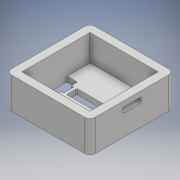
# Autodesk Inventor part: Part4
Saved by Autodesk Inventor 2018 (Build 220112000, 112)
## iProperties
Created: 2019-01-10
Part Number: Part4
Material: Generic
Document SubType Name: Modeling
Designer: USER
Density: 1 g/cm^3
Appearance: Default
Author: USER
Autodesk Inventor part; units mm, degrees
ref_plane "YZ Plane" through (0, 0, 0) normal (1, 0, 0) x (0, 1, 0)
ref_plane "XZ Plane" through (0, 0, 0) normal (0, 1, 0) x (-1, 0, 0)
ref_plane "XY Plane" through (0, 0, 0) normal (0, 0, 1) x (1, 0, 0)
sketch "Sketch1" plane through (0, 0, 0) normal (0, 0, 1) x (1, 0, 0)
  line L0 (-80, -80) -> (80, -80)
  line L1 (80, -80) -> (80, 80)
  line L2 (80, 80) -> (-80, 80)
  line L3 (-80, 80) -> (-80, -80)
  line L4 (-80, -80) -> (80, 80) construction
  line L5 (80, -80) -> (-80, 80) construction
  point P0 (0, 0)
  dimension "d0" = 160
  dimension "d1" = 160
  constraints: 12 end point, 2 midpoint, 2 parallel, 1 horizontal, 1 perpendicular
  measures "d0" distance of L2.end L1.end
  measures "d1" distance of L1.end L0.end
extrude "Extrusion1" add sketch "Sketch1" along normal blind 60
sketch "Sketch2" plane through (0, 0, 60) normal (0, 0, 1) x (1, 0, 0)
  line L0 (-65, 65) -> (65, 65)
  line L1 (65, 65) -> (65, -65)
  line L2 (65, -65) -> (-65, -65)
  line L3 (-65, -65) -> (-65, 65)
  point P0 (0, 0)
  point P1 (-80, 80)
  point P2 (-80, -80)
  point P3 (80, -80)
  constraints: 8 end point, 2 parallel, 1 horizontal, 1 perpendicular
extrude "Extrusion2" cut sketch "Sketch2" against normal blind 50
sketch "Sketch18" plane through (0, 0, 0) normal (0, 0, -1) x (-1, 0, 0)
  line L0 (80, 80) -> (80, -80)
  line L1 (80, 80) -> (80, -80) projected
  line L2 (45, 20) -> (65, 20)
  line L3 (65, 20) -> (65, -20)
  line L4 (65, -20) -> (45, -20)
  line L5 (45, -20) -> (45, 20)
  line L6 (45, 20) -> (65, -20) construction
  line L7 (65, 20) -> (45, -20) construction
  point P0 (0, 0)
  dimension "d40" = 20
  dimension "d41" = 40
  constraints: 14 end point, 2 parallel, 1 horizontal, 1 perpendicular
  measures "d40" distance of L3.end L4.end
  measures "d41" distance of L2.end L3.end
extrude "Extrusion5" cut sketch "Sketch18" against normal blind 20
sketch "Sketch26" plane through (-78, 80, 0) normal (0, 1, 0) x (1, 0, 0)
  line L0 (143, -12) -> (143, -18) projected
  line L1 (143, -15) -> (113, -15)
  line L2 (113, -15) -> (113, -25)
  line L3 (113, -25) -> (143, -25)
  line L4 (143, -25) -> (143, -15)
  point P0 (78, 0)
  dimension "d65" = 30
  dimension "d66" = 10
  constraints: 8 end point, 2 parallel, 1 horizontal, 1 midpoint, 1 perpendicular
  measures "d65" distance of L3.end L2.end
  measures "d66" distance of L2.end L1.end
extrude "Extrusion9" cut sketch "Sketch26" against normal blind 20
fillet "Fillet4" radius 2 4 edges at (65, 72.5, 25) (65, 72.5, 15) (35, 72.5, 25) (35, 72.5, 15)
sketch "Sketch36" plane through (0, 0, 10) normal (0, 0, 1) x (1, 0, 0)
  line L0 (0, -10) -> (35, -10)
  line L1 (35, -10) -> (35, 0)
  line L2 (-35, 10) -> (35, 10)
  line L3 (35, 10) -> (35, -10)
  line L4 (35, -10) -> (-35, -10)
  line L5 (-35, -10) -> (-35, 10)
  line L6 (-35, 10) -> (35, -10) construction
  line L7 (35, 10) -> (-35, -10) construction
  point P0 (0, 0)
  dimension "d75" = 10
  dimension "d76" = 35
  dimension "d77" = 10
  constraints: 16 end point, 2 midpoint, 2 parallel, 2 perpendicular, 1 horizontal
  measures "d75" distance of point (0, 0) L0.start
  measures "d76" distance of L0.start L0.end
  measures "d77" distance of L0.end L1.end
extrude "Extrusion11" cut sketch "Sketch36" against normal blind 20
sketch "Sketch37" plane through (0, 0, 10) normal (0, 0, 1) x (1, 0, 0)
  line L0 (-49.7695, 10) -> (-40.2305, 10)
  line L1 (-40.2305, 10) -> (-40.2305, -10)
  line L2 (-40.2305, -10) -> (-49.7695, -10)
  line L3 (-49.7695, -10) -> (-49.7695, 10)
  line L4 (-45, 20) -> (-45, -20) projected
  line L5 (-49.7695, 10) -> (-40.2305, -10) construction
  line L6 (-40.2305, 10) -> (-49.7695, -10) construction
  point P0 (0, 0)
  point P1 (-45, 0)
  point P2 (-45, 18)
  point P3 (-45, -18)
  constraints: 12 end point, 3 midpoint, 2 parallel, 1 horizontal, 1 perpendicular
extrude "Extrusion12" cut sketch "Sketch37" against normal blind 20
fillet "Fillet6" radius 2 4 edges at (35, 10, 5) (35, -10, 5) (-35, -10, 5) (-35, 10, 5)
fillet "Fillet7" radius 10 4 edges at (80, 80, 30) (-80, 80, 30) (-80, -80, 30) (80, -80, 30)
fillet "Fillet8" radius 2 2 edges at (-40.2305, 10, 5) (-40.2305, -10, 5)
sketch "Sketch46" plane through (0, 0, 10) normal (0, 0, 1) x (1, 0, 0)
  line L0 (-65, 20) -> (-45, 20) projected
  line L1 (-45, 20) -> (-45, 21)
  line L2 (-45, -20) -> (-45, -10) projected
  line L3 (-45, -20) -> (-45, -21)
  line L4 (-45, -21) -> (-65, -21)
  line L5 (-65, -21) -> (-65, -20)
  line L6 (-65, -20) -> (-45, -20)
  line L7 (-45, -20) -> (-45, -21)
  line L8 (-45, 21) -> (-65, 21)
  line L9 (-65, 21) -> (-65, 20)
  line L10 (-65, 20) -> (-45, 20)
  line L11 (-45, 20) -> (-45, 21)
  point P0 (0, 0)
  dimension "d87" = 1
  dimension "d88" = 1
  dimension "d89" = 20
  dimension "d90" = 1
  dimension "d91" = 20
  dimension "d92" = 1
  constraints: 20 end point, 4 parallel, 2 horizontal, 2 perpendicular, 2 vertical
  measures "d87" distance of L0.end L1.end
  measures "d88" distance of L2.start L3.end
  measures "d89" distance of L5.end L6.end
  measures "d90" distance of L4.end L5.end
  measures "d91" distance of L10.end L0.start
  measures "d92" distance of L0.start L8.end
extrude "Extrusion13" cut sketch "Sketch46" against normal blind 10
fillet "Fillet9" radius 2 4 edges at (-45, 21, 5) (-65, 21, 5) (-65, -21, 5) (-45, -21, 5)
sketch "Sketch51" plane through (80, -70, 0) normal (1, 0, 0) x (0, 0, -1)
  line L0 (-60, 5) -> (-60, 135) projected
  line L1 (-60, 70) -> (-45, 70)
  line L2 (-50, 52.5) -> (-40, 52.5)
  line L3 (-40, 52.5) -> (-40, 87.5)
  line L4 (-40, 87.5) -> (-50, 87.5)
  line L5 (-50, 87.5) -> (-50, 52.5)
  line L6 (-50, 52.5) -> (-40, 87.5) construction
  line L7 (-40, 52.5) -> (-50, 87.5) construction
  point P0 (0, 70)
  dimension "d103" = 15
  dimension "d104" = 10
  dimension "d105" = 35
  constraints: 14 end point, 3 midpoint, 2 horizontal, 2 parallel, 1 perpendicular
  measures "d103" distance of L1.start L1.end
  measures "d104" distance of L4.end L3.end
  measures "d105" distance of L3.end L2.end
extrude "Extrusion14" cut sketch "Sketch51" against normal blind 30
fillet "Fillet10" radius 2 4 edges at (72.5, -17.5, 40) (72.5, -17.5, 50) (72.5, 17.5, 40) (72.5, 17.5, 50)
body "Solid1"
